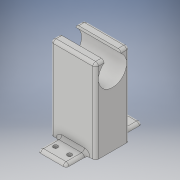
# Autodesk Inventor part: Part2
Saved by Autodesk Inventor 2017 (Build 210142000, 142)
## iProperties
Created: 2016-11-13
Part Number: Part2
Material: Generic
Document SubType Name: Modeling
Designer: Alice
Density: 1 g/cm^3
Appearance: Default
Author: Alice
## iProperties of the stored document Pot_Holder_2_3DPrint.ipt
Created: 2016-11-17
Part Number: Pot_Holder_2_3DPrint
Material: Generic
Document SubType Name: Modeling
Designer: Alice
Density: 1 g/cm^3
Appearance: Default
Author: Alice
Autodesk Inventor part; units mm, degrees
ref_plane "YZ Plane" through (0, 0, 0) normal (1, 0, 0) x (0, 1, 0)
ref_plane "XZ Plane" through (0, 0, 0) normal (0, 1, 0) x (-1, 0, 0)
ref_plane "XY Plane" through (0, 0, 0) normal (0, 0, 1) x (1, 0, 0)
sketch "Sketch1" plane through (0, 0, 0) normal (0, 1, 0) x (-1, 0, 0)
  line L0 (16, -12) -> (-16, -12)
  line L1 (-16, -12) -> (-16, 12)
  line L2 (-16, 12) -> (16, 12)
  line L3 (16, 12) -> (16, -12)
  line L4 (16, -12) -> (-16, 12) construction
  line L5 (-16, -12) -> (16, 12) construction
  line L6 (-10, 27) -> (10, 27)
  line L7 (10, 27) -> (10, -27)
  line L8 (10, -27) -> (-10, -27)
  line L9 (-10, -27) -> (-10, 27)
  line L10 (-10, 27) -> (10, -27) construction
  line L11 (10, 27) -> (-10, -27) construction
  circle A0 centre (5, 19.5) radius 1.5875
  circle A1 centre (5, -19.5) radius 1.5875
  circle A2 centre (-5, 19.5) radius 1.5875
  circle A3 centre (-5, -19.5) radius 1.5875
  point P0 (0, 0)
  dimension "d0" = 32
  dimension "d1" = 24
  dimension "d2" = 20
  dimension "d3" = 54
  dimension "d4" = 3.175
  dimension "d5" = 7.5
  dimension "d7" = 5
  dimension "d10" = 39
  dimension "d13" = 10
  constraints: 24 end point, 4 centre point, 4 midpoint, 4 parallel, 3 horizontal, 2 perpendicular, 1 vertical, 6 other
  measures "d0" distance of L1.end L2.end
  measures "d1" distance of L0.end L1.end
  measures "d2" distance of L7.end L8.end
  measures "d3" distance of L6.end L7.end
  measures "d4" diameter of A0
  measures "d5" distance from line of L6 A0.centre
  measures "d7" distance from line of L7 A0.centre
  measures "d10" distance of A0.centre A1.centre
  measures "d13" distance of A0.centre A2.centre
extrude "Extrusion1" add sketch "Sketch1" along normal blind 2
sketch "Sketch2" plane through (0, 2, 0) normal (0, 1, 0) x (1, 0, 0)
  line L0 (16, 12) -> (16, -12) projected
  line L1 (-16, -12) -> (16, -12)
  line L2 (16, -12) -> (16, 12)
  line L3 (16, 12) -> (-16, 12)
  line L4 (-16, 12) -> (-16, -12)
  line L5 (-16, -12) -> (16, 12) construction
  line L6 (16, -12) -> (-16, 12) construction
  point P0 (0, 0)
  constraints: 12 end point, 2 midpoint, 2 parallel, 1 horizontal, 1 perpendicular
extrude "Extrusion2" add sketch "Sketch2" along normal blind 57.15
sketch "Sketch3" plane through (16, 0, 12) normal (1, 0, 0) x (0, 0, -1)
  line L0 (0, 59.15) -> (24, 59.15) projected
  line L1 (24, 0) -> (0, 0) projected
  line L2 (24, 0) -> (24, 59.15) projected
  line L3 (0, 59.15) -> (24, 59.15) projected
  line L4 (0, 0) -> (0, 59.15) projected
  circle A0 centre (12, 49.15) radius 10
  point P0 (12, 0)
  dimension "d20" = 20
  dimension "d21" = 10
  constraints: 1 centre point
  measures "d20" diameter of A0
  measures "d21" distance from line of L0 A0.centre
extrude "Extrusion3" cut sketch "Sketch3" against normal through all contours A0
sketch "Sketch4" plane through (16, 0, 12) normal (1, 0, 0) x (0, 0, -1)
  circle A0 centre (12, 49.15) radius 10 projected
  line L0 (0, 59.15) -> (12, 59.15) projected
  line L1 (12, 59.15) -> (24, 59.15) projected
  line L2 (12, 59.15) -> (0, 59.15) projected
  line L3 (6, 59.15) -> (18, 59.15)
  line L4 (18, 59.15) -> (18, 57.15)
  line L5 (18, 57.15) -> (6, 57.15)
  line L6 (6, 57.15) -> (6, 59.15)
  point P0 (12, 0)
  constraints: 8 end point, 2 parallel, 1 horizontal, 1 midpoint, 1 perpendicular, 1 point on circle
extrude "Extrusion4" cut sketch "Sketch4" against normal through all contours L5 A0 | A0 L1 L4 | L6 L0 A0 picked at (10.6135, 57.5146)
fillet "Fillet1" radius 2 1 edges at (0, 59.15, 12)
fillet "Fillet2" radius 2 1 edges at (0, 59.15, -12)
fillet "Fillet3" radius 2 3 edges at (16, 58.5642, 11.4142) (16, 59.15, 8) (16, 28.575, 12)
fillet "Fillet4" radius 2 3 edges at (16, 58.5642, -11.4142) (16, 59.15, -8) (16, 28.575, -12)
fillet "Fillet5" radius 2 1 edges at (10, 1, 27)
fillet "Fillet6" radius 2 1 edges at (10, 1, -27)
fillet "Fillet7" radius 2 1 edges at (-10, 1, 27)
fillet "Fillet8" radius 2 1 edges at (-10, 1, -27)
fillet "Fillet9" radius 2 3 edges at (-16, 28.575, -12) (-16, 58.5642, -11.4142) (-16, 59.15, -8)
fillet "Fillet10" radius 2 3 edges at (-16, 28.575, 12) (-16, 58.5642, 11.4142) (-16, 59.15, 8)
fillet "Fillet11" radius 2 5 edges at (10, 2, 18.5) (9.4142, 2, 26.4142) (0, 2, 27) (-9.4142, 2, 26.4142) (-10, 2, 18.5)
fillet "Fillet12" radius 2 3 edges at (0, 2, 12) (-9.4144, 1.4144, 12) (9.4144, 1.4144, 12)
fillet "Fillet13" radius 2 5 edges at (0, 2, -27) (-9.4142, 2, -26.4142) (-10, 2, -18.5) (9.4142, 2, -26.4142) (10, 2, -18.5)
fillet "Fillet14" radius 2 3 edges at (0, 2, -12) (9.4144, 1.4144, -12) (-9.4144, 1.4144, -12)
body "Solid1"
